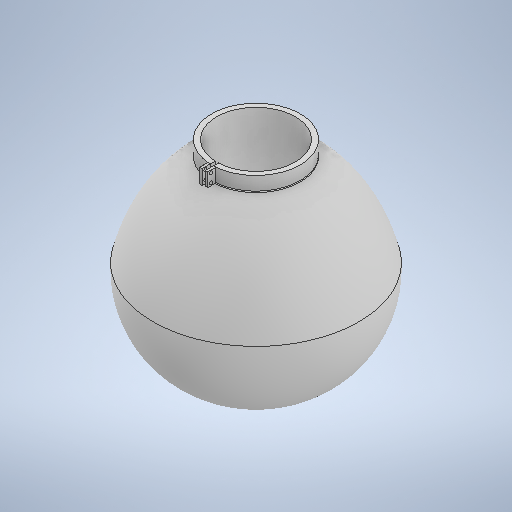
# Autodesk Inventor part: Water Sensor Bouy
Saved by Autodesk Inventor 2025 (Build 290162000, 162)
## iProperties
Created: 2024-06-17
Part Number: Water Sensor Bouy
Material: Generic
Document SubType Name: Modeling
Designer: track
Density: 1 g/cm^3
Appearance: Default
Mass: 1114.84 g
Surface Area: 2537.18 cm^2
Volume: 1114.84 cm^3
Author: track
## iProperties of the stored document Water Sensor Bouy_3DPrint.ipt
Created: 2024-06-17
Part Number: Water Sensor Bouy_3DPrint
Material: Generic
Document SubType Name: Modeling
Designer: track
Density: 1 g/cm^3
Appearance: Default
Author: track
Autodesk Inventor part; units mm, degrees
ref_plane "YZ Plane" through (0, 0, 0) normal (1, 0, 0) x (0, 1, 0)
sketch "Sketch1" plane through (0, 0, 0) normal (0, 0, 1) x (1, 0, 0)
  line L0 (0, 0) -> (0, 76.2)
  line L1 (31.2895, 0) -> (31.2895, 152.4)
  line L2 (31.2895, 76.2) -> (82.0895, 76.2)
  arc A0 (82.0895, 76.2) -> (31.2895, 152.4) centre (-41.8733, 48.5915) ccw
  arc A1 (31.2895, 0) -> (82.0895, 76.2) centre (6.0118, 71.8852) ccw
  line L3 (32.2895, 150.4536) -> (32.2895, 1.4258)
  arc A2 (32.2895, 1.4258) -> (81.0957, 76.0622) centre (6.0118, 71.8852) ccw
  arc A3 (81.0957, 76.0622) -> (32.2895, 150.4536) centre (-41.8733, 48.5915) ccw
  point P0 (31.2895, 50.8)
  dimension "d1" = 31.2895
  dimension "d3" = 0
  dimension "d74" = 152.4
  dimension "d75" = 50.8
  dimension "d76" = 76.2
  dimension "d78" = 127
  dimension "d83" = 1
  dimension "d129" = 76.2
  dimension "d187" = 126
  dimension "d188" = 73.1628
  constraints: 8 end point, 8 point on circle, 4 centre point, 2 vertical, 1 horizontal, 1 midpoint, 1 point on line, 2 other
  measures "d1" distance between parallel lines of L1 L0
  measures "d3" vertical distance of L0.start L1.start
  measures "d74" distance of L1.start L1.end
  measures "d75" distance of L2.start L2.end
  measures "d76" distance from line of L1.end L2
  measures "d78" radius of A0
  measures "d83" distance between parallel lines of L1 L3
  measures "d129" radius of A1
  measures "d187" radius of A3
  measures "d188" horizontal distance of L1.start A0.centre
revolve "Revolution1" add sketch "Sketch1" angle 360 about axis through (0, 0, 0) along (0, 1, 0) contours L1 L2 L3 A2 A3 A1 | L1 A0 L2 A3 L3
sketch "Sketch27" plane through (0, 0, 0) normal (0, 1, 0) x (-1, 0, 0)
  line L0 (0, 0) -> (-82.0895, 0)
  circle A0 centre (0, 0) radius 82.0895 projected
  circle A1 centre (-50.8, 0) radius 3.175
  dimension "d150" = 6.35
  dimension "d151" = 50.8
  constraints: 2 end point, 1 centre point, 1 horizontal, 1 horizontal alignment, 1 point on line, 1 other
  measures "d150" diameter of A1
  measures "d151" distance of L0.start A1.centre
extrude "Extrusion18" cut sketch "Sketch27" along normal blind 33.02 contours A1 L0 | L0 A1
pattern_circular "Circular Pattern5" count 3 over 360 about axis through (0, 71.8852, 0) along (0, 1, 0) of "Extrusion18"
ref_plane "Work Plane7" through (0, 152.4, 0) normal (0, 1, 0) x (-1, 0, 0)
sketch "Sketch39" plane through (0, 152.4, 0) normal (0, 1, 0) x (-1, 0, 0)
  circle A0 centre (0, 0) radius 31.2895
  circle A1 centre (0, 0) radius 31.2895 projected
  circle A2 centre (0, 0) radius 35.2895
  dimension "d190" = 4
  constraints: 2 centre point, 1 coincident, 1 concentric
  measures "d190" radial gap between concentric circles of A0 A2
extrude "Extrusion25" add sketch "Sketch39" along normal blind 8.89 and the other way blind 4
ref_plane "Work Plane8" through (0, 152.4, 35.2895) normal (0, 0, 1) x (1, 0, 0)
sketch "Sketch41" plane through (0, 152.4, 35.2895) normal (0, 0, 1) x (1, 0, 0)
  line L0 (-35.2895, -2.9378) -> (35.2895, -2.9378) projected
  line L1 (-31.2895, 8.89) -> (31.2895, 8.89) projected
  line L2 (-3.27, -2.9378) -> (-1.27, -2.9378)
  line L3 (-1.27, -2.9378) -> (-1.27, 8.89)
  line L4 (-1.27, 8.89) -> (-3.27, 8.89)
  line L5 (-3.27, 8.89) -> (-3.27, -2.9378)
  line L6 (1.27, -2.9378) -> (3.27, -2.9378)
  line L7 (3.27, -2.9378) -> (3.27, 8.89)
  line L8 (3.27, 8.89) -> (1.27, 8.89)
  line L9 (1.27, 8.89) -> (1.27, -2.9378)
  line L10 (0, 8.89) -> (0, -2.9378)
  point P0 (0, -152.4)
  point P1 (-3.27, 8.89)
  point P2 (1.27, 8.89)
  point P3 (1.27, -2.9378)
  dimension "d195" = 2.54
  dimension "d196" = 2
  constraints: 18 end point, 4 parallel, 4 point on line, 2 horizontal, 2 midpoint, 2 perpendicular, 2 other
  measures "d195" distance between parallel lines of L3 L9
  measures "d196" distance between parallel lines of L9 L7
extrude "Extrusion26" add sketch "Sketch41" along normal blind 6.35 contours L5 L1 L3 L0 | L9 L1 L7 L0
sketch "Sketch42" plane through (0, 152.4, 41.6395) normal (0, 0, 1) x (1, 0, 0)
  line L0 (-1.27, -2.9378) -> (-1.27, 8.89) projected
  line L1 (1.27, -2.9378) -> (3.27, -2.9378) projected
  line L2 (-1.27, 8.89) -> (1.27, 8.89)
  line L3 (1.27, 8.89) -> (1.27, -2.9378)
  line L4 (1.27, -2.9378) -> (-1.27, -2.9378)
  line L5 (-1.27, -2.9378) -> (-1.27, 8.89)
  line L6 (1.27, -1.9378) -> (35.2895, -1.9378)
  line L7 (35.2895, -1.9378) -> (35.2895, -2.9378)
  line L8 (35.2895, -2.9378) -> (1.27, -2.9378)
  line L9 (1.27, -2.9378) -> (1.27, -1.9378)
  line L10 (35.2895, 8.89) -> (-35.2895, 8.89) projected
  line L11 (35.2895, 8.89) -> (35.2895, -2.9378)
  arc A0 (82.0895, -76.2) -> (35.2895, -2.9378) centre (-41.8733, -103.8085) ccw projected
  point P0 (0, -152.4)
  point P1 (0, 8.89)
  dimension "d200" = 0
  dimension "d201" = 1
  constraints: 18 end point, 4 parallel, 2 horizontal, 2 perpendicular, 2 point on line, 1 midpoint, 1 point on circle, 1 vertical
  measures "d200" distance between parallel lines of L11 L7
  measures "d201" distance between parallel lines of L8 L6
extrude "Extrusion27" cut sketch "Sketch42" against normal blind 63.5 contours L0 L2 L3 L4 | L3 L6 L7 L8 L1
sketch "Sketch43" plane through (3.27, 161.29, 41.6395) normal (1, 0, 0) x (0, 0, -1)
  line L0 (6.35, 0) -> (0, 0) projected
  line L1 (2.54, 0) -> (2.54, -10.8278)
  line L2 (6.35, -10.8278) -> (0, -10.8278) projected
  line L3 (0, -10.8278) -> (0, 0) projected
  circle A0 centre (2.54, -1.905) radius 1.27
  circle A1 centre (2.54, -8.9228) radius 1.27
  point P0 (41.6395, -161.29)
  dimension "d204" = 2.54
  dimension "d205" = 2.54
  dimension "d206" = 2.54
  dimension "d207" = 1.905
  dimension "d208" = 1.905
  constraints: 4 point on line, 2 centre point, 2 end point, 1 vertical
  measures "d204" distance between parallel lines of L3 L1
  measures "d205" diameter of A0
  measures "d206" diameter of A1
  measures "d207" distance from line of L2 A1.centre
  measures "d208" distance from line of L0 A0.centre
extrude "Extrusion28" cut sketch "Sketch43" against normal up to surface (6.54 mm away) contours A0 L1 | L1 A0 | A1 L1 | L1 A1
body "Solid1"
